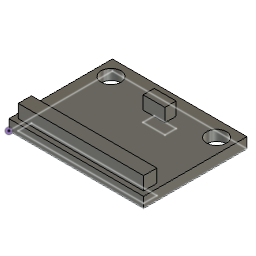
MP6050 (Autodesk Fusion 360 design; units mm, degrees)
Autodesk Fusion 360 part; units mm, degrees
sketch "Sketch1" plane through (0, 0, 0) normal (0, 0, 1) x (1, 0, 0)
  line L0 (0, 0) -> (20.3, 0)
  line L1 (20.3, 0) -> (20.3, 15.6)
  line L2 (20.3, 15.6) -> (0, 15.6)
  line L3 (0, 15.6) -> (0, 0)
  line L4 (9, 12.9) -> (12.3, 12.9)
  line L5 (12.3, 12.9) -> (12.3, 11.22)
  line L6 (12.3, 11.22) -> (9, 11.22)
  line L7 (9, 11.22) -> (9, 12.9)
  line L8 (0.7, 2.7) -> (19.6, 2.7)
  line L9 (19.6, 2.7) -> (19.6, 0.7)
  line L10 (19.6, 0.7) -> (0.7, 0.7)
  line L11 (0.7, 0.7) -> (0.7, 2.7)
  dimension "d1" = 20.3
  dimension "d2" = 15.6
  dimension "d3" = 3.3
  dimension "d4" = 1.68
  dimension "d5" = 2.7
  dimension "d6" = 8
  dimension "d7" = 0.7
  dimension "d8" = 2
  dimension "d9" = 0.7
  dimension "d10" = 0.7
  constraint horizontal L0
  constraint vertical L1
  constraint horizontal L2
  constraint vertical L3
  constraint coincident L0.start L3.end
  constraint horizontal L4
  constraint vertical L5
  constraint horizontal L6
  constraint vertical L7
  constraint horizontal L8
  constraint vertical L9
  constraint horizontal L10
  constraint vertical L11
  measures "d1" distance of L0.start L0.end
  measures "d2" distance of L0.start L2.end
  measures "d3" distance of L4.start L4.end
  measures "d4" distance of L4.start L6.end
  measures "d5" distance of L2 L4
  measures "d6" distance of L1 L5
  measures "d7" distance of L0 L10
  measures "d8" distance of L8 L10
  measures "d9" distance of L3 L11
  measures "d10" distance of L1 L9
extrude "Extrude1" add sketch "Sketch1" along normal blind 1.6 contours L0 L1 L2 L3 | L4 L5 L6 L7 | L8 L9 L10 L11
extrude "Extrude2" add sketch "Sketch1" along normal blind 3.6 contours L4 L5 L6 L7
extrude "Extrude3" add sketch "Sketch1" along normal blind 3.6 and the other way blind 0.5 contours L8 L9 L10 L11
sketch "Sketch2" plane through (0, 0, 1.6) normal (0, 0, 1) x (-1, 0, 0)
  line L0 (-0.7, -0.7) -> (-0.7, -2.7)
  line L1 (-0.7, -2.7) -> (-19.6, -2.7)
  line L2 (-19.6, -2.7) -> (-19.6, -0.7)
  line L3 (-19.6, -0.7) -> (-0.7, -0.7)
  line L4 (-9, -11.22) -> (-9, -12.9)
  line L5 (-9, -12.9) -> (-12.3, -12.9)
  line L6 (-12.3, -12.9) -> (-12.3, -11.22)
  line L7 (-12.3, -11.22) -> (-9, -11.22)
  line L8 (0, -15.6) -> (0, 0)
  line L9 (0, 0) -> (-20.3, 0)
  line L10 (-20.3, 0) -> (-20.3, -15.6)
  line L11 (-20.3, -15.6) -> (0, -15.6)
  circle A0 centre (-2.2, -13.2) radius 1.5
  line L12 (-20.3, -15.6) -> (0, -15.6)
  line L13 (0, -15.6) -> (0, 0)
  line L14 (-10.15, -15.6) -> (-10.15, -9.9904) construction
  circle A1 centre (-18.1, -13.2) radius 1.5
  dimension "d19" = 3
  dimension "d21" = 2.4
  dimension "d22" = 2.2
  constraint midpoint L11 L14.start
  constraint perpendicular L12 L14
  constraint symmetric A0 L14 A1
  measures "d19" diameter of A0
  measures "d21" distance of A0.centre L12
  measures "d22" distance of A0.centre L13
extrude "Extrude4" cut sketch "Sketch2" against normal through all contours A0 | A1
equation "d21 = 0.9 mm + ( d19 / 2 )"
equation "d22 = 0.7 mm + ( d19 / 2 )"
